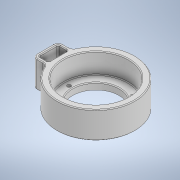
# Autodesk Inventor part: front_hip_motor_protector
Saved by Autodesk Inventor 2020.2 (Build 242310000, 310)
## iProperties
Created: 2021-02-08
Part Number: front_hip_motor_protector
Material: Generic
Document SubType Name: Modeling
Designer: DELL
Density: 1 g/cm^3
Appearance: Default
Author: DELL
Autodesk Inventor part; units mm, degrees
ref_plane "YZ Plane" through (0, 0, 0) normal (1, 0, 0) x (0, 1, 0)
ref_plane "XZ Plane" through (0, 0, 0) normal (0, 1, 0) x (-1, 0, 0)
ref_plane "XY Plane" through (0, 0, 0) normal (0, 0, 1) x (1, 0, 0)
sketch "Sketch1" plane through (0, 0, 0) normal (0, 1, 0) x (-1, 0, 0)
  circle A0 centre (0, 0) radius 48
  circle A1 centre (0, 0) radius 40
  circle A2 centre (0, 0) radius 28.5
  circle A3 centre (0, 0) radius 33 construction
  line L0 (0, 0) -> (16.5, 28.5788) construction
  line L1 (48, 0) -> (-48, 0) construction
  circle A4 centre (33, 0) radius 2.25
  circle A5 centre (16.5, 28.5788) radius 2.25
  circle A6 centre (33, 0) radius 3.75
  circle A7 centre (16.5, 28.5788) radius 3.75
  line L2 (0, 48) -> (0, -48) construction
  circle A8 centre (16.5, -28.5788) radius 2.25
  circle A9 centre (16.5, -28.5788) radius 3.75
  circle A10 centre (-16.5, 28.5788) radius 2.25
  circle A11 centre (-16.5, 28.5788) radius 3.75
  circle A12 centre (-16.5, -28.5788) radius 3.75
  circle A13 centre (-16.5, -28.5788) radius 2.25
  line L3 (0, 0) -> (-16.5, 28.5788) construction
  line L4 (-20, 34.641) -> (2.9783, 47.9075)
  line L5 (-16.5, 28.5788) -> (-20, 34.641) construction
  line L6 (-20, -34.641) -> (2.9783, -47.9075)
  line L7 (46.4758, 12) -> (58.4758, 12)
  line L8 (58.4758, 12) -> (58.4758, -12)
  line L9 (58.4758, -12) -> (46.4758, -12)
  line L10 (45.2548, -16) -> (62.4758, -16)
  line L11 (62.4758, -16) -> (62.4758, 16)
  line L12 (62.4758, 16) -> (45.2548, 16)
  line L13 (46.4758, -12) -> (46.4758, 12)
  point P0 (2.9783, -47.9075)
  dimension "d0" = 96
  dimension "d1" = 80
  dimension "d2" = 57
  dimension "d3" = 66
  dimension "d4" = 60
  dimension "d5" = 4.5
  dimension "d6" = 7.5
  dimension "d16" = 24
  dimension "d18" = 4
  dimension "d21" = 10.4758
  dimension "d34" = 12
  dimension "d35" = 32
  dimension "d36" = 17.221
  constraints: 28 end point, 13 centre point, 10 coincident, 8 symmetric about line, 4 point on circle, 3 horizontal, 3 midpoint, 2 equal radius, 2 perpendicular, 2 point on line, 2 vertical, 1 collinear, 1 tangent, 21 other
  measures "d1" diameter of A1
  measures "d2" diameter of A2
  measures "d3" diameter of A3
  measures "d4" angle of L1 L0
  measures "d5" diameter of A4
  measures "d6" diameter of A6
  measures "d16" distance between parallel lines of L7 L9
  measures "d18" distance between parallel lines of L11 L8
  measures "d21" distance from line of L1.start L8
  measures "d34" distance between parallel lines of L13 L8
  measures "d35" distance between parallel lines of L12 L10
  measures "d36" distance of L11.end L12.end
extrude "Extrusion1" add sketch "Sketch1" along normal blind 8 contours L13 A0 L6 A1 L4 | L4 A1 L6 A0 | A1 | A5 | A6 | A7 | A8 | A9 | A11 | A12
extrude "Extrusion2" add sketch "Sketch1" along normal blind 25 from surface at 8 contours L13 A0 L6 A1 L4 | L4 A1 L6 A0
extrude "Extrusion3" cut sketch "Sketch1" along normal blind 3 contours A4 | A6 | A10 | A11 | A12 | A13
fillet "Fillet1" [suppressed]
fillet "Fillet2" [suppressed]
extrude "Extrusion5" add sketch "Sketch1" along normal up to surface (33 mm away) contours A0 L12 L11 L10 L9 L8 L7
fillet "Fillet4" radius 6 4 edges at (-45.2548, 16.5, 16) (-45.2548, 16.5, -16) (-62.4758, 16.5, -16) (-62.4758, 16.5, 16)
fillet "Fillet5" radius 2 4 edges at (-46.4758, 16.5, -12) (-58.4758, 16.5, -12) (-58.4758, 16.5, 12) (-46.4758, 16.5, 12)
fillet "Fillet3" radius 1 21 edges at (-20, 8, 34.641) (48, 33, 0) (-20, 33, 34.641) (48, 0, 0) (28.5, 8, 0) (-57.89, 33, -11.4142) (-58.4758, 33, 0) (-57.89, 33, 11.4142) (-52.4758, 33, 12) (-47.0616, 33, 11.4142) (-46.4758, 33, 0) (-47.0616, 33, -11.4142) (-52.4758, 33, -12) (-47.0616, 0, 11.4142) (-52.4758, 0, 12) (-57.89, 0, 11.4142) (-58.4758, 0, 0) (-57.89, 0, -11.4142) (-52.4758, 0, -12) (-47.0616, 0, -11.4142) (-46.4758, 0, 0)
equation "\"hole\" = 1.8"
equation "\"wall\" = 0.6"
body "Solid1"
body "Solid2"
body "Solid3"
body "Solid4"
body "Solid5"
